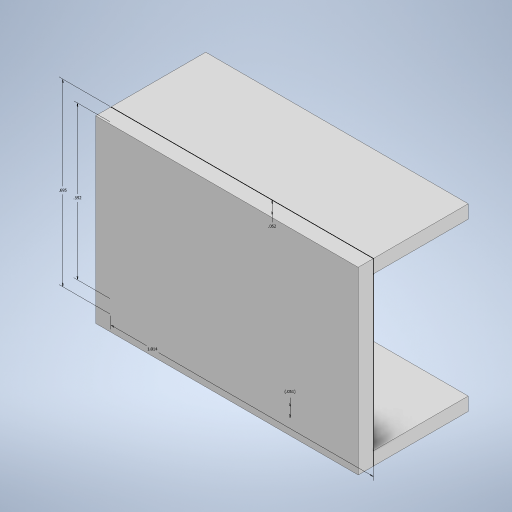
# Autodesk Inventor part: Cover
Saved by Autodesk Inventor 2024 (Build 280153000, 153)
## iProperties
Created: 2024-04-29
Part Number: Cover
Material: Generic
Document SubType Name: Modeling
Designer: Hitesh
Density: 1 g/cm^3
Appearance: Default
Author: Hitesh
Autodesk Inventor part; units mm, degrees
ref_plane "YZ Plane" through (0, 0, 0) normal (1, 0, 0) x (0, 1, 0)
ref_plane "XZ Plane" through (0, 0, 0) normal (0, 1, 0) x (-1, 0, 0)
ref_plane "XY Plane" through (0, 0, 0) normal (0, 0, 1) x (1, 0, 0)
sketch "Sketch1" plane through (0, 0, 0) normal (0, 0, 1) x (1, 0, 0)
  line L0 (0, 17.6499) -> (25.7669, 17.6499)
  line L1 (25.7669, 17.6499) -> (25.7669, 0)
  line L2 (25.7669, 0) -> (0, 0)
  line L3 (0, 0) -> (0, 17.6499)
  line L4 (25.7669, 17.6499) -> (0, 17.6499)
  line L5 (0, 17.6499) -> (0, 16.3405)
  line L6 (0, 16.3405) -> (25.7669, 16.3405)
  line L7 (25.7669, 16.3405) -> (25.7669, 17.6499)
  line L8 (25.7669, 0) -> (0, 0)
  line L9 (0, 0) -> (0, 1.306)
  line L10 (0, 1.306) -> (25.7669, 1.306)
  line L11 (25.7669, 1.306) -> (25.7669, 0)
  dimension "d0" = 17.65
  dimension "d1" = 15.0345
  dimension "d2" = 1.3094
  dimension "d3" = 1.306
  dimension "d4" = 25.7669
  constraints: 24 end point, 6 parallel, 3 horizontal, 3 perpendicular, 2 point on line, 1 coincident
  measures "d0" distance between parallel lines of L2 L0
  measures "d1" distance between parallel lines of L10 L6
  measures "d2" distance between parallel lines of L6 L0
  measures "d3" distance between parallel lines of L2 L10
  measures "d4" distance of L1.end L2.end
extrude "Extrusion1" add sketch "Sketch1" along normal blind 1.5
extrude "Extrusion2" add sketch "Sketch1" against normal blind 9.3 contours L0 L1 L6 L3 | L10 L1 L2 L3
body "Solid1"
